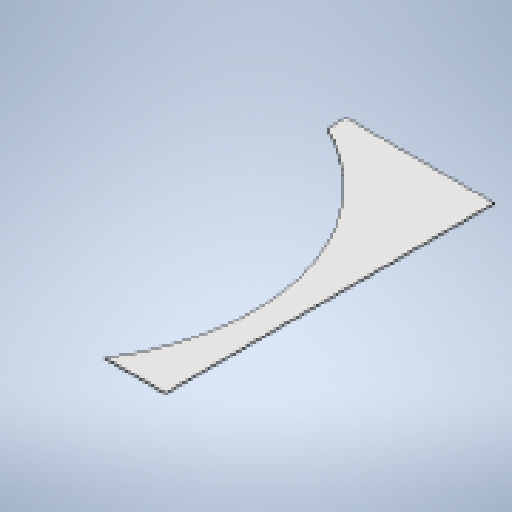
# Autodesk Inventor part: TRM 013 top main
Saved by Autodesk Inventor 2025 (Build 290162010, 162A)
## iProperties
Created: 2024-08-07
Part Number: TRM 013 top main
Material: AISI 304
Document SubType Name: Sheet Metal
Designer: pokla
Density: 8.02768 g/cm^3
Flat Pattern Width: 22.5813 cm
Flat Pattern Length: 50.2864 cm
Flat Pattern Area: 1135.53 cm^2
Sheet Metal Rule: AISI304 2mm Die16
Sheet Metal Width: 225,813 mm
Sheet Metal Length: 502,864 mm
Sheet Metal Area: 113553,396 mm^2
Appearance: Default
Stock Number: ТРМ 013 верх основное
Author: pokla
Autodesk Inventor part; units mm, degrees
ref_plane "YZ Plane" through (0, 0, 0) normal (1, 0, 0) x (0, 1, 0)
ref_plane "XZ Plane" through (0, 0, 0) normal (0, 1, 0) x (-1, 0, 0)
ref_plane "XY Plane" through (0, 0, 0) normal (0, 0, 1) x (1, 0, 0)
sketch "Sketch1" plane through (0, 0, 0) normal (0, 0, 1) x (1, 0, 0)
  line L0 (-112.9066, -251.4321) -> (112.9066, -251.4321)
  line L1 (112.9066, -251.4321) -> (112.9066, 251.4321)
  line L2 (112.9066, 251.4321) -> (-112.9066, 251.4321)
  line L3 (-112.9066, 251.4321) -> (-112.9066, -251.4321)
  line L4 (-112.9066, -251.4321) -> (112.9066, 251.4321) construction
  line L5 (112.9066, -251.4321) -> (-112.9066, 251.4321) construction
  arc A0 (20.3035, -251.4321) -> (-112.9066, 222.3681) centre (-257.2283, -73.8346) ccw
  point P0 (0, 0)
extrude "Plate1" add sketch "Sketch1" along normal blind 2 contours A0 L3 L2 L1 L0
sketch "Sketch2" plane through (0, 0, 0) normal (0, 0, -1) x (-1, 0, 0)
  line L0 (-92.9066, 231.4321) -> (107.0934, 231.4321) construction
  line L1 (107.0934, 231.4321) -> (107.0934, 211.4321) construction
  line L2 (107.0934, 211.4321) -> (-92.9066, 211.4321) construction
  line L3 (-92.9066, 211.4321) -> (-92.9066, 231.4321) construction
  line L4 (-112.9066, 251.4321) -> (112.9066, 251.4321) projected
  line L5 (-112.9066, -251.4321) -> (-112.9066, 251.4321) projected
  point P0 (0, 0)
  dimension "d6" = 200
  dimension "d9" = 20
  dimension "d10" = 20
  dimension "d11" = 20
  constraints: 2 other
  measures "d6" distance of L0.start L0.end
  measures "d9" distance of L0.end L1.end
  measures "d10" distance between parallel lines of L4 L0
  measures "d11" distance between parallel lines of L5 L3
mark "Mark1"
equation "\"d2\" = Thickness"
equation "\"BendReliefWidth\" = Thickness"
equation "\"BendReliefDepth\" = 0.5 * Thickness"
equation "\"CornerReliefSize\" = 4 * Thickness"
equation "\"MinimumRemnant\" = 2 * Thickness"
equation "\"TransitionRadius\" = BendRadius"
equation "\"JacobiRadiusSize\" = BendRadius"
equation "\"GapSize\" = Thickness"
equation "\"Thickness\" = 2"
equation "\"BendRadius\" = 2.75"
body "Solid1"
